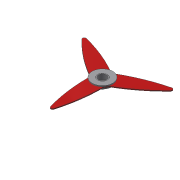
# Autodesk Inventor part: Wind Turbine Propeller
Saved by Autodesk Inventor 2015 SP1 (Build 190203100, 203)
## iProperties
Created: 2015-08-24
Part Number: Wind Turbine Propeller
Material: 一般
Document SubType Name: Modeling
Designer: nobuhiro
Density: 1 g/cm^3
Appearance: 既定
Author: nobuhiro
Autodesk Inventor part; units mm, degrees
ref_plane "YZ Plane" through (0, 0, 0) normal (1, 0, 0) x (0, 1, 0)
ref_plane "XZ Plane" through (0, 0, 0) normal (0, 1, 0) x (-1, 0, 0)
ref_plane "XY Plane" through (0, 0, 0) normal (0, 0, 1) x (1, 0, 0)
sketch "スケッチ1" plane through (0, 0, 0) normal (0, 0, 1) x (1, 0, 0)
  circle A0 centre (0, 0) radius 28.5
  circle A1 centre (0, 0) radius 60
  arc A2 (9.6165, -292.7429) -> (45, -39.6863) centre (-877.5991, -39.6863) ccw
  arc A3 (-9.6165, -292.7429) -> (9.6165, -292.7429) centre (0, -290) ccw
  arc A4 (-45, -39.6863) -> (-9.6165, -292.7429) centre (877.5991, -39.6863) ccw
  circle A5 centre (0, 0) radius 300 construction
  line L0 (45, -39.6863) -> (45, -370.5857) construction
  line L1 (45, -370.5857) -> (-45, -370.5857) construction
  line L2 (-45, -370.5857) -> (-45, -39.6863) construction
  circle A6 centre (0, 0) radius 28.5
  circle A7 centre (0, 0) radius 60
  arc A8 (248.7145, 154.6995) -> (11.8693, 58.8143) centre (473.1689, -740.1799) ccw
  arc A9 (258.331, 138.0433) -> (248.7145, 154.6995) centre (251.1474, 145) ccw
  arc A10 (56.8693, -19.128) -> (258.331, 138.0433) centre (-404.4302, 779.8663) ccw
  circle A11 centre (0, 0) radius 28.5
  circle A12 centre (0, 0) radius 60
  arc A13 (-258.331, 138.0433) -> (-56.8693, -19.128) centre (404.4302, 779.8663) ccw
  arc A14 (-248.7145, 154.6995) -> (-258.331, 138.0433) centre (-251.1474, 145) ccw
  arc A15 (-11.8693, 58.8143) -> (-248.7145, 154.6995) centre (-473.1689, -740.1799) ccw
  point P0 (11.8693, 58.8143)
  point P1 (56.8693, -19.128)
  point P2 (-56.8693, -19.128)
  point P3 (-11.8693, 58.8143)
  dimension "d1" = 90
  dimension "d2" = 600
  dimension "d3" = 120
  dimension "d4" = 57
  dimension "d5" = 90
  dimension "d7" = 10
  dimension "d10" = 360
  constraints: 30 point on circle, 16 centre point, 11 coincident, 6 end point, 5 tangent, 2 vertical, 1 equal radius, 1 horizontal alignment, 1 perpendicular, 1 vertical alignment, 53 other
  measures "d1" distance of A1.end A1.start
  measures "d2" diameter of A5
  measures "d3" diameter of A1
  measures "d4" diameter of A0
  measures "d5" distance of L0.end L1.end
  measures "d7" radius of A3
extrude "押し出し1" add sketch "スケッチ1" along normal mid plane 5
sketch "スケッチ3" plane through (0, 0, 0) normal (0, 1, 0) x (-1, 0, 0)
  line L0 (28.5, -2.5) -> (-28.5, -2.5) projected
  line L1 (28.5, 8.5) -> (28.5, -19)
  line L2 (28.5, -19) -> (24, -19)
  line L3 (24, -19) -> (24, 8.5)
  line L4 (24, 8.5) -> (28.5, 8.5)
  line L5 (0, 0) -> (0, -47.5) construction
  arc A0 (0, -47.5) -> (28.5, -19) centre (0, -19) ccw
  arc A1 (0, -43) -> (24, -19) centre (0, -19) ccw
  line L6 (0, -47.5) -> (0, -43)
  line L7 (45, 2.5) -> (9.6165, 2.5) projected
  dimension "d17" = 24
  dimension "d18" = 28.5
  dimension "d19" = 45
  dimension "d24" = 6
  constraints: 12 end point, 4 perpendicular, 4 point on circle, 3 vertical, 2 centre point, 2 tangent, 1 point on line, 1 vertical alignment
  measures "d17" distance between parallel lines of L5 L3
  measures "d18" distance between parallel lines of L5 L1
  measures "d19" distance from line of L0 L5.end
  measures "d24" distance between parallel lines of L7 L4
revolve "回転1" add sketch "スケッチ3" angle 360 about axis through (0, 0, 0) along (0, 0, -1)
sketch "スケッチ4" plane through (0, 0, 2.5) normal (0, 0, 1) x (1, 0, 0)
  circle A0 centre (0, 0) radius 28.5 projected
  arc A1 (-56.8693, -19.128) -> (-45, -39.6863) centre (0, 0) ccw projected
  circle A2 centre (0, 0) radius 60
  constraints: 1 coincident, 3 other
extrude "押し出し3" add sketch "スケッチ4" along normal blind 6 and the other way blind 11 separate body
